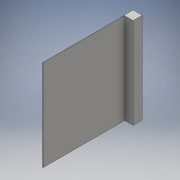
# Autodesk Inventor part: Ecran_Videoprojecteur
Saved by Autodesk Inventor 2016 SP1 (Build 200210100, 210)
## iProperties
Created: 2016-10-06
Part Number: Ecran_Videoprojecteur
Material: Générique
Document SubType Name: Modeling
Designer: dimercur
Density: 1 g/cm^3
Appearance: Par défaut
Author: dimercur
Autodesk Inventor part; units mm, degrees
ref_plane "YZ Plane" through (0, 0, 0) normal (1, 0, 0) x (0, 1, 0)
ref_plane "XZ Plane" through (0, 0, 0) normal (0, 1, 0) x (-1, 0, 0)
ref_plane "XY Plane" through (0, 0, 0) normal (0, 0, 1) x (1, 0, 0)
sketch "Esquisse1" plane through (0, 0, 0) normal (0, 0, 1) x (1, 0, 0)
  line L0 (-100, 100) -> (100, 100)
  line L1 (100, 100) -> (100, -100)
  line L2 (100, -100) -> (-100, -100)
  line L3 (-100, -100) -> (-100, 100)
  line L4 (-95.2971, -100) -> (-85.2971, -100)
  line L5 (-85.2971, -100) -> (-85.2971, -1900)
  line L6 (-85.2971, -1900) -> (-95.2971, -1900)
  line L7 (-95.2971, -1900) -> (-95.2971, -100)
  point P0 (0, 0)
  dimension "d0" = 200
  dimension "d1" = 200
  dimension "d2" = 100
  dimension "d3" = 100
  dimension "d4" = 1800
  dimension "d5" = 10
  constraints: 16 end point, 4 parallel, 2 horizontal, 2 perpendicular, 1 point on line
  measures "d0" distance of L0.start L0.end
  measures "d1" distance of L2.end L0.start
  measures "d2" horizontal distance of point (0, 0) L0.start
  measures "d3" horizontal distance of point (0, 0) L0.start
  measures "d4" distance of L6.end L4.start
  measures "d5" distance of L5.end L6.end
extrude "Extrusion1" add sketch "Esquisse1" along normal blind 2000
sketch "Esquisse2" plane through (-100, 100, 0) normal (0, 1, 0) x (1, 0, 0)
  line L0 (14.7029, 0) -> (14.7029, -2000) projected
  line L1 (14.7029, -1926.0048) -> (14.7029, -1942.8259)
  line L2 (4.7029, 0) -> (4.7029, -2000) projected
  line L3 (4.7029, -126.1575) -> (4.7029, -105.1313)
  line L4 (0, 0) -> (0, -2000) projected
  line L5 (0, -1900) -> (-100, -1900)
  line L6 (-100, -1900) -> (-100, -1885)
  line L7 (-100, -1885) -> (0, -1885)
  line L8 (0, -1885) -> (0, -1900)
  line L9 (0, -115) -> (-100, -115)
  line L10 (-100, -115) -> (-100, -100)
  line L11 (-100, -100) -> (0, -100)
  line L12 (0, -100) -> (0, -115)
  point P0 (100, 0)
  dimension "d8" = 100
  dimension "d9" = 15
  dimension "d10" = 100
  dimension "d11" = 100
  dimension "d12" = 15
  dimension "d13" = 100
  constraints: 20 end point, 4 parallel, 4 point on line, 2 horizontal, 2 perpendicular
  measures "d8" distance of L9.start L9.end
  measures "d9" distance of L9.end L10.end
  measures "d10" distance from line of L4.start L11
  measures "d11" distance from line of L5 L4.end
  measures "d12" distance of L5.end L6.end
  measures "d13" distance of L6.end L7.end
extrude "Extrusion2" add sketch "Esquisse2" against normal blind 150
sketch "Esquisse3" plane through (-200, 100, 1900) normal (0, 0, 1) x (1, 0, 0)
  line L0 (0, -150) -> (100, -150) projected
  line L1 (100, 0) -> (100, -200) projected
  line L2 (15, -150) -> (100, -150)
  line L3 (100, -150) -> (100, -15)
  line L4 (100, -15) -> (15, -15)
  line L5 (15, -15) -> (15, -150)
  line L6 (0, 0) -> (100, 0) projected
  point P0 (200, -100)
  dimension "d16" = 15
  dimension "d17" = 15
  constraints: 8 end point, 2 parallel, 2 point on line, 1 horizontal, 1 perpendicular
  measures "d16" distance between parallel lines of L6 L4
  measures "d17" distance of L2.start L0.start
extrude "Extrusion3" cut sketch "Esquisse3" against normal through all
equation "\"d2\" = 0.5 * d1"
equation "\"d3\" = 0.5 * d0"
